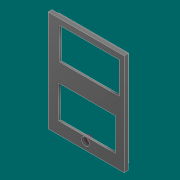
# Autodesk Inventor part: tappo_superiore
Saved by Autodesk Inventor 2020 (Build 240168000, 168)
## iProperties
Created: 2025-02-23
Part Number: tappo_superiore
Material: Plastica ABS
Document SubType Name: Modeling
Designer: Nicola Milia
Density: 1.06 g/cm^3
Appearance: Liscia - Bianco
Author: Nicola Milia
## iProperties of the stored document _Stampa 3D.ipt
Created: 2025-02-23
Part Number: _Stampa 3D
Material: Generico
Document SubType Name: Modeling
Designer: Nicola Milia
Density: 1 g/cm^3
Appearance: Default
Author: Nicola Milia
Autodesk Inventor part; units mm, degrees
ref_plane "YZ Plane" through (0, 0, 0) normal (1, 0, 0) x (0, 1, 0)
ref_plane "XZ Plane" through (0, 0, 0) normal (0, 1, 0) x (-1, 0, 0)
ref_plane "XY Plane" through (0, 0, 0) normal (0, 0, 1) x (1, 0, 0)
ref_plane "Piano di lavoro1" through (0, 0, 0) normal (0, 0, 1) x (1, 0, 0)
sketch "Schizzo1" plane through (0, 0, 0) normal (0, 0, 1) x (1, 0, 0)
  line L0 (42, 19.3) -> (42, 54.3) projected
  line L1 (42, 54.3) -> (-33, 54.3) projected
  line L2 (-33, 54.3) -> (-33, 19.3) projected
  line L3 (-33, 19.3) -> (42, 19.3) projected
  line L4 (38, -13) -> (-35, -13) projected
  line L5 (-35, -13) -> (-35, -48) projected
  line L6 (-35, -48) -> (38, -48) projected
  line L7 (38, -48) -> (38, -13) projected
  line L8 (45.5, 61.5) -> (45.5, -61.5) projected
  line L9 (-45.5, 61.5) -> (45.5, 61.5) projected
  line L10 (45.5, -61.5) -> (-45.5, -61.5) projected
  line L11 (-45.5, -61.5) -> (-45.5, 61.5) projected
  line L12 (-48.5, -64.5) -> (48.5, -64.5) projected
  line L13 (-48.5, 64.5) -> (-48.5, -64.5) projected
  line L14 (48.5, -64.5) -> (48.5, 64.5) projected
  line L15 (48.5, 64.5) -> (-48.5, 64.5) projected
  line L16 (-45, -61) -> (45, -61) projected
  line L17 (45, -61) -> (-1, -61)
  line L18 (-1, -61) -> (-1, -55)
  circle A0 centre (-1, -55) radius 5
  line L19 (43.5, -59.5) -> (43.5, 59.5)
  line L20 (43.5, 59.5) -> (-43.5, 59.5)
  line L21 (-43.5, 59.5) -> (-43.5, -59.5)
  line L22 (-43.5, -59.5) -> (43.5, -59.5)
  point P0 (0, 0)
  point P1 (-3.1794, -59.5)
  point P2 (1.1794, -59.5)
  dimension "d0" = 46
  dimension "d1" = 6
  dimension "d2" = 10
  dimension "d3" = 2
  constraints: 12 end point, 1 centre point, 1 coincident, 1 perpendicular, 1 point on line, 3 other
  measures "d0" distance of L16.end L17.end
  measures "d1" distance of L17.end L18.end
  measures "d2" diameter of A0
  measures "d3" distance between parallel lines of L8 L19
ref_plane "Piano di lavoro2" through (0, 0, 0) normal (0, 0, 1) x (1, 0, 0)
sketch "Schizzo2" plane through (0, 0, 0) normal (0, 0, 1) x (1, 0, 0)
  line L0 (-48.5, 64.5) -> (-48.5, -64.5) projected
  circle A0 centre (-1, -55) radius 5 projected
  line L1 (45.5, 61.5) -> (45.5, -61.5) projected
  point P0 (0, 0)
extrude "Estrusione1" add sketch "Schizzo1" against normal blind 5 contours L8 L10 L11 L9
ref_plane "Piano di lavoro3" through (0, 0, 0) normal (0, 0, 1) x (1, 0, 0)
sketch "Schizzo3" plane through (0, 0, 0) normal (0, 0, 1) x (1, 0, 0)
  line L0 (-48.5, 64.5) -> (-48.5, -64.5) projected
  line L1 (48.5, 64.5) -> (-48.5, 64.5) projected
  line L2 (48.5, -64.5) -> (48.5, 64.5) projected
  line L3 (-48.5, -64.5) -> (48.5, -64.5) projected
  circle A0 centre (-1, -55) radius 5 projected
  point P0 (0, 0)
extrude "Estrusione2" add sketch "Schizzo3" along normal blind 5
sketch "Schizzo4" plane through (0, 0, 5) normal (0, 0, 1) x (1, 0, 0)
  circle A0 centre (-1, -55) radius 5 projected
  line L0 (-35, -48) -> (38, -48) projected
  line L1 (38, -48) -> (38, -13) projected
  line L2 (38, -13) -> (-35, -13) projected
  line L3 (-35, -13) -> (-35, -48) projected
  line L4 (42, 19.3) -> (42, 54.3) projected
  line L5 (-33, 19.3) -> (42, 19.3) projected
  line L6 (-33, 54.3) -> (-33, 19.3) projected
  line L7 (42, 54.3) -> (-33, 54.3) projected
  point P0 (0, 0)
extrude "Estrusione3" cut sketch "Schizzo4" against normal up to surface (5 mm away)
move faces "Sposta1" translate (0, 0, 2.5) faces at (15.6667, 8.5333, 0)
move faces "Sposta2" translate (0, 2.75, 0) faces at (17, 54.3, 4.1667)
move faces "Sposta3" translate (0, -2.75, 0) faces at (-8, 19.3, 4.1667)
move faces "Sposta4" translate (0, 2.75, 0) faces at (13.6667, -13, 4.1667)
move faces "Sposta5" translate (0, -1, 0) faces at (-10.6667, -48, 4.1667)
move faces "Sposta6" translate (0, 1, 0) faces at (13.6667, -10.25, 4.1667)
thicken "Ispessimento1" operation add thickness 1 both sides no extend neighbours yes toward (0, 1, 0) faces at (-15.1667, -61.5, -1.6667) (-45.5, 20.5, -1.6667) (45.5, -20.5, -1.6667) (15.1667, 61.5, -1.6667)
move faces "Sposta7" translate (-1, 0, 0) faces at (-33, 42.6333, 4.1667) (-33, 55.2167, 4.1667) (-33, 17.4667, 4.1667)
move faces "Sposta8" translate (0, 2, 0) faces at (13.6667, -9.25, 4.1667)
